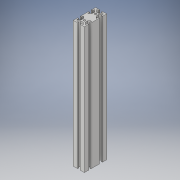
# Autodesk Inventor part: 1530rail_17inch
Saved by Autodesk Inventor 2018 (Build 220112000, 112)
## iProperties
Created: 2020-03-10
Part Number: 1530rail_17inch
Material: Generic
Document SubType Name: Modeling
Designer: natha
Density: 1 g/cm^3
Appearance: Default
Author: natha
Autodesk Inventor part; units mm, degrees
ref_plane "YZ Plane" through (0, 0, 0) normal (1, 0, 0) x (0, 1, 0)
ref_plane "XZ Plane" through (0, 0, 0) normal (0, 1, 0) x (-1, 0, 0)
ref_plane "XY Plane" through (0, 0, 0) normal (0, 0, 1) x (1, 0, 0)
sketch "Sketch1" plane through (0, 0, 0) normal (0, 1, 0) x (-1, 0, 0)
  circle A0 centre (19.05, -19.05) radius 3.3274
  circle A1 centre (19.05, -57.15) radius 3.3274
  line L0 (0, 0) -> (15.0114, 0)
  line L1 (15.0114, 0) -> (15.0114, -4.2672)
  line L2 (15.0114, -4.2672) -> (8.001, -4.2672)
  line L3 (38.1, 0) -> (23.0886, 0)
  line L4 (23.0886, 0) -> (23.0886, -4.2672)
  line L5 (23.0886, -4.2672) -> (30.099, -4.2672)
  line L6 (23.0886, -11.0548) -> (15.0114, -11.0548)
  line L7 (30.099, -4.2672) -> (23.0886, -11.0548)
  line L8 (8.001, -4.2672) -> (15.0114, -11.0548)
  line L9 (38.1, 0) -> (38.1, -15.0114)
  line L10 (38.1, -15.0114) -> (33.8328, -15.0114)
  line L11 (33.8328, -15.0114) -> (33.8328, -8.001)
  line L12 (38.1, -76.2) -> (38.1, -61.1886)
  line L13 (38.1, -61.1886) -> (33.8328, -61.1886)
  line L14 (33.8328, -61.1886) -> (33.8328, -68.199)
  line L15 (38.1, -76.2) -> (23.0886, -76.2)
  line L16 (23.0886, -76.2) -> (23.0886, -71.9328)
  line L17 (23.0886, -71.9328) -> (30.099, -71.9328)
  line L18 (38.1, -23.0124) -> (38.1, -52.2224)
  line L19 (38.1, -23.0124) -> (33.8328, -23.0124)
  line L20 (33.8328, -23.0124) -> (33.8328, -30.0228)
  line L21 (38.1, -52.2224) -> (33.8328, -52.2224)
  line L22 (33.8328, -52.2224) -> (33.8328, -45.212)
  line L23 (26.1112, -15.0114) -> (26.1112, -23.0124)
  line L24 (26.1112, -52.2224) -> (26.1112, -61.1886)
  line L25 (33.8328, -8.001) -> (26.1112, -15.0114)
  line L26 (26.1112, -23.0124) -> (33.8328, -30.0228)
  line L27 (33.8328, -45.212) -> (26.1112, -52.2224)
  line L28 (26.1112, -61.1886) -> (33.8328, -68.199)
  line L29 (0, -76.2) -> (15.0114, -76.2)
  line L30 (15.0114, -76.2) -> (15.0114, -71.9328)
  line L31 (15.0114, -71.9328) -> (8.001, -71.9328)
  line L32 (23.0886, -64.2112) -> (15.0114, -64.2112)
  line L33 (15.0114, -64.2112) -> (8.001, -71.9328)
  line L34 (30.099, -71.9328) -> (23.0886, -64.2112)
  line L35 (0, 0) -> (0, -15.0114)
  line L36 (0, -15.0114) -> (4.2672, -15.0114)
  line L37 (4.2672, -15.0114) -> (4.2672, -8.001)
  line L38 (0, -76.2) -> (0, -61.1886)
  line L39 (0, -61.1886) -> (4.2672, -61.1886)
  line L40 (4.2672, -61.1886) -> (4.2672, -68.199)
  line L41 (11.9888, -15.0114) -> (11.9888, -23.0886)
  line L42 (11.9888, -15.0114) -> (4.2672, -8.001)
  line L43 (0, -22.3774) -> (0, -51.5874)
  line L44 (0, -51.5874) -> (4.2672, -51.5874)
  line L45 (4.2672, -51.5874) -> (4.2672, -44.577)
  line L46 (0, -22.3774) -> (4.2672, -22.3774)
  line L47 (4.2672, -22.3774) -> (4.2672, -29.3878)
  line L48 (4.2672, -29.3878) -> (11.9888, -23.0886)
  line L49 (11.9888, -61.1886) -> (11.9888, -53.1114)
  line L50 (4.2672, -68.199) -> (11.9888, -61.1886)
  line L51 (11.9888, -53.1114) -> (4.2672, -44.577)
  dimension "d0" = 38.1
  dimension "d1" = 76.2
  dimension "d2" = 6.6548
  dimension "d3" = 6.6548
  dimension "d8" = 15.0114
  dimension "d9" = 4.2672
  dimension "d10" = 7.0104
  dimension "d11" = 15.0114
  dimension "d12" = 4.2672
  dimension "d13" = 7.0104
  dimension "d14" = 15.0114
  dimension "d15" = 4.2672
  dimension "d16" = 7.0104
  dimension "d17" = 15.0114
  dimension "d18" = 4.2672
  dimension "d19" = 7.0104
  dimension "d20" = 15.0114
  dimension "d21" = 4.2672
  dimension "d22" = 7.0104
  dimension "d23" = 29.21
  dimension "d24" = 7.0104
  dimension "d25" = 4.2672
  dimension "d26" = 7.0104
  dimension "d27" = 8.001
  dimension "d28" = 11.9888
  dimension "d29" = 8.9662
  dimension "d32" = 11.9888
  dimension "d33" = 15.0114
  dimension "d34" = 4.2672
  dimension "d35" = 7.0104
  dimension "d36" = 11.9888
  dimension "d37" = 76.2
  dimension "d38" = 15.0114
  dimension "d39" = 4.2672
  dimension "d40" = 90
  dimension "d41" = 7.0104
  dimension "d42" = 15.0114
  dimension "d43" = 7.0104
  dimension "d44" = 8.0772
  dimension "d45" = 11.9888
  dimension "d46" = 29.21
  dimension "d47" = 7.0104
  dimension "d48" = 7.0104
  dimension "d49" = 8.0772
  dimension "d50" = 11.9888
  constraints: 104 end point, 20 perpendicular, 10 horizontal, 10 vertical, 2 centre point
  measures "d0" distance of L12.start L29.start
  measures "d1" distance of L3.start L12.start
  measures "d2" diameter of A0
  measures "d3" diameter of A1
  measures "d8" distance of L0.start L0.end
  measures "d9" distance of L0.end L1.end
  measures "d10" distance of L1.end L2.end
  measures "d11" distance of L3.start L3.end
  measures "d12" distance of L3.end L4.end
  measures "d13" distance of L4.end L5.end
  measures "d14" distance of L3.start L9.end
  measures "d15" distance of L9.end L10.end
  measures "d16" distance of L10.end L11.end
  measures "d17" distance of L12.start L12.end
  measures "d18" distance of L12.end L13.end
  measures "d19" distance of L13.end L14.end
  measures "d20" distance of L12.start L15.end
  measures "d21" distance of L15.end L16.end
  measures "d22" distance of L16.end L17.end
  measures "d23" distance of L18.start L18.end
  measures "d24" distance of L19.end L20.end
  measures "d25" distance of L18.end L21.end
  measures "d26" distance of L21.end L22.end
  measures "d27" distance between parallel lines of L19 L10
  measures "d28" distance between parallel lines of L9 L23
  measures "d29" distance of L24.start L24.end
  measures "d32" distance between parallel lines of L9 L24
  measures "d33" distance of L29.start L29.end
  measures "d34" distance of L29.end L30.end
  measures "d35" distance of L30.end L31.end
  measures "d36" distance between parallel lines of L29 L32
  measures "d37" distance of L29.start L0.start
  measures "d38" distance of L0.start L35.end
  measures "d39" distance of L35.end L36.end
  measures "d40" angle of L36 L35
  measures "d41" distance of L36.end L37.end
  measures "d42" distance of L29.start L38.end
  measures "d43" distance of L39.end L40.end
  measures "d44" distance of L41.start L41.end
  measures "d45" distance between parallel lines of L41 L35
  measures "d46" distance of L43.start L43.end
  measures "d47" distance of L44.end L45.end
  measures "d48" distance of L46.end L47.end
  measures "d49" distance of L49.start L49.end
  measures "d50" distance between parallel lines of L38 L49
extrude "Extrusion1" add sketch "Sketch1" along normal blind 431.8
body "Solid1"
